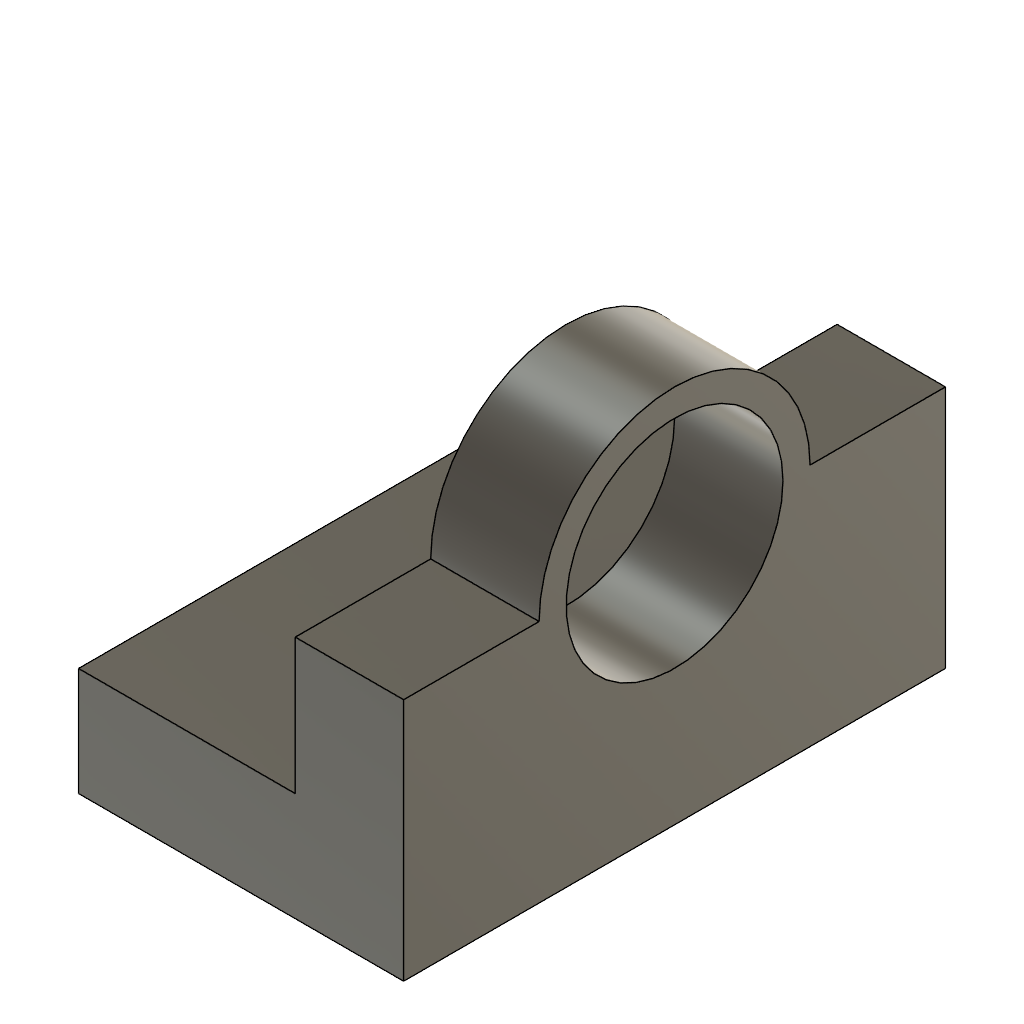
exercise 3 (Autodesk Fusion 360 design; units mm, degrees)
part number: 2026-10-01-22-38-48-408
Autodesk Fusion 360 part; units mm, degrees
note: some values were not read from the file. Set by a fixed rule: which sketch regions a step uses.
sketch "Sketch1" plane through (0, 0, 0) normal (0, 1, 0) x (1, 0, 0)
  line L0 (0, 0) -> (0, -45)
  line L1 (0, -45) -> (-20, -45)
  line L2 (-20, -45) -> (-20, -20)
  line L3 (-20, -20) -> (-60, -20)
  line L4 (-60, -20) -> (-60, 0)
  line L5 (-60, 0) -> (0, 0)
  dimension "d1" = 60
  dimension "d2" = 45
  dimension "d3" = 20
  dimension "d4" = 20
  constraint coincident L0.start L5.end
  constraint vertical L0
  constraint perpendicular L0 L1
  constraint perpendicular L1 L2
  constraint perpendicular L2 L3
  constraint perpendicular L3 L4
  constraint perpendicular L0 L5
  measures "d1" distance of L0.start L4.end
  measures "d2" distance of L0.start L0.end
  measures "d3" distance of L3.end L4.end
  measures "d4" distance of L0.end L1.end
extrude "Extrude1" add sketch "Sketch1" along normal blind 100
sketch "Sketch2" plane through (-20, 0, 0) normal (-1, 0, 0) x (0, -1, 0)
  line L0 (0, 20) -> (0, 45)
  line L1 (0, 45) -> (-100, 45)
  line L2 (-100, 45) -> (-100, 20)
  line L3 (-100, 20) -> (0, 20)
  arc A0 (-25, 45) -> (-75, 45) centre (-50, 45) ccw
  circle A1 centre (-50, 45) radius 20
  dimension "d7" = 50
  dimension "d8" = 40
  constraint midpoint L1 A0.centre
  constraint coincident L1 A0.start
  constraint coincident L1 A0.end
  constraint concentric A0 A1
  measures "d7" diameter of A0
  measures "d8" diameter of A1
extrude "Extrude2" cut sketch "Sketch2" against normal blind 25.469 contours L1 A1 | L1 A1
extrude "Extrude3" add sketch "Sketch2" against normal blind 20 contours L1 A0 A1
